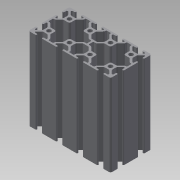
# Autodesk Inventor part: 25-5010
Saved by Autodesk Inventor 2013 (Build 170138000, 138)
## iProperties
Created: 2014-04-23
Part Number: 25-5010
Material: Generic
Document SubType Name: Modeling
Designer: Ross Bowman
Density: 1 g/cm^3
Engineer: Ross Bowman
Catalog Web Link: 8020.net
Vendor: 80/20 Inc.
Company: 80/20 Inc.
Author: Ross Bowman
Keywords: 80/20 , 8020 , T-Slot , Extrusion
Material: 6105-T5 Aluminum
Autodesk Inventor part; units mm, degrees
ref_plane "YZ Plane" through (0, 0, 0) normal (1, 0, 0) x (0, 1, 0)
ref_plane "XZ Plane" through (0, 0, 0) normal (0, 1, 0) x (-1, 0, 0)
ref_plane "XY Plane" through (0, 0, 0) normal (0, 0, 1) x (1, 0, 0)
sketch "Sketch1" plane through (0, 0, 0) normal (0, 0, 1) x (1, 0, 0)
  circle A0 centre (12.5003, -12.5001) radius 2.5
  circle A1 centre (37.5003, -12.5001) radius 2.5
  circle A2 centre (12.5003, 12.4999) radius 2.5
  circle A3 centre (37.5003, 12.4999) radius 2.5
  arc A4 (27.9491, 21.8456) -> (28.8746, 19.6112) centre (31.1091, 21.8456) ccw
  line L0 (32.3392, 16.1466) -> (28.8746, 19.6112)
  arc A5 (32.9878, 14.5807) -> (32.3392, 16.1466) centre (30.7732, 14.5807) ccw
  line L1 (32.9878, 10.1953) -> (32.9878, 14.5807)
  arc A6 (32.9878, 10.1953) -> (35.2024, 7.9807) centre (35.2024, 10.1953) ccw
  line L2 (39.5877, 7.9807) -> (35.2024, 7.9807)
  arc A7 (41.1537, 7.3321) -> (39.5877, 7.9807) centre (39.5877, 5.7661) ccw
  line L3 (44.6183, 3.8675) -> (41.1537, 7.3321)
  arc A8 (44.6183, 3.8675) -> (46.8527, 2.942) centre (46.8527, 6.102) ccw
  line L4 (47.1082, 2.942) -> (46.8527, 2.942)
  arc A9 (47.8588, 2.1914) -> (47.1082, 2.942) centre (47.1082, 2.1914) ccw
  line L5 (47.8588, -2.1939) -> (47.8588, 2.1914)
  arc A10 (47.1082, -2.9445) -> (47.8588, -2.1939) centre (47.1082, -2.1939) ccw
  line L6 (46.8527, -2.9445) -> (47.1082, -2.9445)
  arc A11 (46.8527, -2.9445) -> (44.6183, -3.8701) centre (46.8527, -6.1045) ccw
  line L7 (41.1537, -7.3346) -> (44.6183, -3.8701)
  arc A12 (39.5877, -7.9833) -> (41.1537, -7.3346) centre (39.5877, -5.7687) ccw
  line L8 (35.2024, -7.9833) -> (39.5877, -7.9833)
  arc A13 (35.2024, -7.9833) -> (32.9878, -10.1979) centre (35.2024, -10.1979) ccw
  line L9 (32.9878, -14.5832) -> (32.9878, -10.1979)
  arc A14 (32.3392, -16.1491) -> (32.9878, -14.5832) centre (30.7732, -14.5832) ccw
  line L10 (28.8746, -19.6137) -> (32.3392, -16.1491)
  arc A15 (28.8746, -19.6137) -> (27.9491, -21.8482) centre (31.1091, -21.8482) ccw
  line L11 (27.9491, -22.1036) -> (27.9491, -21.8482)
  arc A16 (27.1985, -22.8542) -> (27.9491, -22.1036) centre (27.1985, -22.1036) ccw
  line L12 (22.8132, -22.8542) -> (27.1985, -22.8542)
  arc A17 (22.0626, -22.1036) -> (22.8132, -22.8542) centre (22.8132, -22.1036) ccw
  line L13 (22.0626, -21.8482) -> (22.0626, -22.1036)
  arc A18 (22.0626, -21.8482) -> (21.137, -19.6137) centre (18.9026, -21.8482) ccw
  line L14 (17.6725, -16.1491) -> (21.137, -19.6137)
  arc A19 (17.0238, -14.5832) -> (17.6725, -16.1491) centre (19.2384, -14.5832) ccw
  line L15 (17.0238, -10.1979) -> (17.0238, -14.5832)
  arc A20 (17.0238, -10.1979) -> (14.8092, -7.9833) centre (14.8092, -10.1979) ccw
  line L16 (10.4239, -7.9833) -> (14.8092, -7.9833)
  arc A21 (8.8579, -7.3346) -> (10.4239, -7.9833) centre (10.4239, -5.7687) ccw
  line L17 (5.3934, -3.8701) -> (8.8579, -7.3346)
  arc A22 (5.3934, -3.8701) -> (3.1589, -2.9445) centre (3.1589, -6.1045) ccw
  line L18 (1.8176, -2.9445) -> (3.1589, -2.9445)
  arc A23 (1.067, -2.1939) -> (1.8176, -2.9445) centre (1.8176, -2.1939) ccw
  line L19 (1.067, 2.1914) -> (1.067, -2.1939)
  arc A24 (1.8176, 2.942) -> (1.067, 2.1914) centre (1.8176, 2.1914) ccw
  line L20 (3.1589, 2.942) -> (1.8176, 2.942)
  arc A25 (3.1589, 2.942) -> (5.3934, 3.8675) centre (3.1589, 6.102) ccw
  line L21 (8.8579, 7.3321) -> (5.3934, 3.8675)
  arc A26 (10.4239, 7.9807) -> (8.8579, 7.3321) centre (10.4239, 5.7661) ccw
  line L22 (14.8092, 7.9807) -> (10.4239, 7.9807)
  arc A27 (14.8092, 7.9807) -> (17.0238, 10.1953) centre (14.8092, 10.1953) ccw
  line L23 (17.0238, 14.5807) -> (17.0238, 10.1953)
  arc A28 (17.6725, 16.1466) -> (17.0238, 14.5807) centre (19.2384, 14.5807) ccw
  line L24 (21.137, 19.6112) -> (17.6725, 16.1466)
  arc A29 (21.137, 19.6112) -> (22.0626, 21.8456) centre (18.9026, 21.8456) ccw
  line L25 (22.0626, 22.1011) -> (22.0626, 21.8456)
  arc A30 (22.8132, 22.8517) -> (22.0626, 22.1011) centre (22.8132, 22.1011) ccw
  line L26 (27.1985, 22.8517) -> (22.8132, 22.8517)
  arc A31 (27.9491, 22.1011) -> (27.1985, 22.8517) centre (27.1985, 22.1011) ccw
  line L27 (27.9491, 21.8456) -> (27.9491, 22.1011)
  arc A32 (-2.9417, -21.8482) -> (-3.8673, -19.6137) centre (-6.1017, -21.8482) ccw
  line L28 (-7.0501, -16.4309) -> (-3.8673, -19.6137)
  arc A33 (-7.9756, -14.1965) -> (-7.0501, -16.4309) centre (-4.8156, -14.1965) ccw
  line L29 (-7.9756, -10.8104) -> (-7.9756, -14.1965)
  arc A34 (-7.0501, -8.5759) -> (-7.9756, -10.8104) centre (-4.8156, -10.8104) ccw
  line L30 (-3.8673, -5.3931) -> (-7.0501, -8.5759)
  arc A35 (-3.1559, -5.0984) -> (-3.8673, -5.3931) centre (-3.1559, -6.1045) ccw
  line L31 (3.1589, -5.0984) -> (-3.1559, -5.0984)
  arc A36 (3.8703, -5.3931) -> (3.1589, -5.0984) centre (3.1589, -6.1045) ccw
  line L32 (7.0531, -8.5759) -> (3.8703, -5.3931)
  arc A37 (7.9787, -10.8104) -> (7.0531, -8.5759) centre (4.8187, -10.8104) ccw
  line L33 (7.9787, -14.1965) -> (7.9787, -10.8104)
  arc A38 (7.0531, -16.4309) -> (7.9787, -14.1965) centre (4.8187, -14.1965) ccw
  line L34 (3.8703, -19.6137) -> (7.0531, -16.4309)
  arc A39 (3.8703, -19.6137) -> (2.9448, -21.8482) centre (6.1048, -21.8482) ccw
  line L35 (2.9448, -22.1036) -> (2.9448, -21.8482)
  arc A40 (2.1942, -22.8542) -> (2.9448, -22.1036) centre (2.1942, -22.1036) ccw
  line L36 (-2.1911, -22.8542) -> (2.1942, -22.8542)
  arc A41 (-2.9417, -22.1036) -> (-2.1911, -22.8542) centre (-2.1911, -22.1036) ccw
  line L37 (-2.9417, -21.8482) -> (-2.9417, -22.1036)
  circle A42 centre (-12.5003, -12.5001) radius 2.5
  circle A43 centre (-37.5003, -12.5001) radius 2.5
  arc A44 (-3.8673, 19.6112) -> (-2.9417, 21.8456) centre (-6.1017, 21.8456) ccw
  line L38 (-2.9417, 22.1011) -> (-2.9417, 21.8456)
  arc A45 (-2.1911, 22.8517) -> (-2.9417, 22.1011) centre (-2.1911, 22.1011) ccw
  line L39 (2.1942, 22.8517) -> (-2.1911, 22.8517)
  arc A46 (2.9448, 22.1011) -> (2.1942, 22.8517) centre (2.1942, 22.1011) ccw
  line L40 (2.9448, 21.8456) -> (2.9448, 22.1011)
  arc A47 (2.9448, 21.8456) -> (3.8703, 19.6112) centre (6.1048, 21.8456) ccw
  line L41 (7.0531, 16.4284) -> (3.8703, 19.6112)
  arc A48 (7.9787, 14.1939) -> (7.0531, 16.4284) centre (4.8187, 14.1939) ccw
  line L42 (7.9787, 10.8078) -> (7.9787, 14.1939)
  arc A49 (7.0531, 8.5734) -> (7.9787, 10.8078) centre (4.8187, 10.8078) ccw
  line L43 (3.8703, 5.3906) -> (7.0531, 8.5734)
  arc A50 (3.1589, 5.0959) -> (3.8703, 5.3906) centre (3.1589, 6.102) ccw
  line L44 (-3.1559, 5.0959) -> (3.1589, 5.0959)
  arc A51 (-3.8673, 5.3906) -> (-3.1559, 5.0959) centre (-3.1559, 6.102) ccw
  line L45 (-7.0501, 8.5734) -> (-3.8673, 5.3906)
  arc A52 (-7.9756, 10.8078) -> (-7.0501, 8.5734) centre (-4.8156, 10.8078) ccw
  line L46 (-7.9756, 14.1939) -> (-7.9756, 10.8078)
  arc A53 (-7.0501, 16.4284) -> (-7.9756, 14.1939) centre (-4.8156, 14.1939) ccw
  line L47 (-3.8673, 19.6112) -> (-7.0501, 16.4284)
  circle A54 centre (-12.5003, 12.4999) radius 2.5
  circle A55 centre (-37.5003, 12.4999) radius 2.5
  arc A56 (-28.8716, 19.6112) -> (-27.946, 21.8456) centre (-31.106, 21.8456) ccw
  line L48 (-27.946, 22.1011) -> (-27.946, 21.8456)
  arc A57 (-27.1954, 22.8517) -> (-27.946, 22.1011) centre (-27.1954, 22.1011) ccw
  line L49 (-22.8101, 22.8517) -> (-27.1954, 22.8517)
  arc A58 (-22.0595, 22.1011) -> (-22.8101, 22.8517) centre (-22.8101, 22.1011) ccw
  line L50 (-22.0595, 21.8456) -> (-22.0595, 22.1011)
  arc A59 (-22.0595, 21.8456) -> (-21.134, 19.6112) centre (-18.8995, 21.8456) ccw
  line L51 (-17.6694, 16.1466) -> (-21.134, 19.6112)
  arc A60 (-17.0208, 14.5807) -> (-17.6694, 16.1466) centre (-19.2354, 14.5807) ccw
  line L52 (-17.0208, 10.1953) -> (-17.0208, 14.5807)
  arc A61 (-17.0208, 10.1953) -> (-14.8062, 7.9807) centre (-14.8062, 10.1953) ccw
  line L53 (-10.4208, 7.9807) -> (-14.8062, 7.9807)
  arc A62 (-8.8549, 7.3321) -> (-10.4208, 7.9807) centre (-10.4208, 5.7661) ccw
  line L54 (-5.3903, 3.8675) -> (-8.8549, 7.3321)
  arc A63 (-5.3903, 3.8675) -> (-3.1559, 2.942) centre (-3.1559, 6.102) ccw
  line L55 (-1.8146, 2.942) -> (-3.1559, 2.942)
  arc A64 (-1.064, 2.1914) -> (-1.8146, 2.942) centre (-1.8146, 2.1914) ccw
  line L56 (-1.064, -2.1939) -> (-1.064, 2.1914)
  arc A65 (-1.8146, -2.9445) -> (-1.064, -2.1939) centre (-1.8146, -2.1939) ccw
  line L57 (-3.1559, -2.9445) -> (-1.8146, -2.9445)
  arc A66 (-3.1559, -2.9445) -> (-5.3903, -3.8701) centre (-3.1559, -6.1045) ccw
  line L58 (-8.8549, -7.3346) -> (-5.3903, -3.8701)
  arc A67 (-10.4208, -7.9833) -> (-8.8549, -7.3346) centre (-10.4208, -5.7687) ccw
  line L59 (-14.8062, -7.9833) -> (-10.4208, -7.9833)
  arc A68 (-14.8062, -7.9833) -> (-17.0208, -10.1979) centre (-14.8062, -10.1979) ccw
  line L60 (-17.0208, -14.5832) -> (-17.0208, -10.1979)
  arc A69 (-17.6694, -16.1491) -> (-17.0208, -14.5832) centre (-19.2354, -14.5832) ccw
  line L61 (-21.134, -19.6137) -> (-17.6694, -16.1491)
  arc A70 (-21.134, -19.6137) -> (-22.0595, -21.8482) centre (-18.8995, -21.8482) ccw
  line L62 (-22.0595, -22.1036) -> (-22.0595, -21.8482)
  arc A71 (-22.8101, -22.8542) -> (-22.0595, -22.1036) centre (-22.8101, -22.1036) ccw
  line L63 (-27.1954, -22.8542) -> (-22.8101, -22.8542)
  arc A72 (-27.946, -22.1036) -> (-27.1954, -22.8542) centre (-27.1954, -22.1036) ccw
  line L64 (-27.946, -21.8482) -> (-27.946, -22.1036)
  arc A73 (-27.946, -21.8482) -> (-28.8716, -19.6137) centre (-31.106, -21.8482) ccw
  line L65 (-32.3361, -16.1491) -> (-28.8716, -19.6137)
  arc A74 (-32.9848, -14.5832) -> (-32.3361, -16.1491) centre (-30.7702, -14.5832) ccw
  line L66 (-32.9848, -10.1979) -> (-32.9848, -14.5832)
  arc A75 (-32.9848, -10.1979) -> (-35.1994, -7.9833) centre (-35.1994, -10.1979) ccw
  line L67 (-39.5847, -7.9833) -> (-35.1994, -7.9833)
  arc A76 (-41.1506, -7.3346) -> (-39.5847, -7.9833) centre (-39.5847, -5.7687) ccw
  line L68 (-44.6152, -3.8701) -> (-41.1506, -7.3346)
  arc A77 (-44.6152, -3.8701) -> (-46.8497, -2.9445) centre (-46.8497, -6.1045) ccw
  line L69 (-47.1051, -2.9445) -> (-46.8497, -2.9445)
  arc A78 (-47.8557, -2.1939) -> (-47.1051, -2.9445) centre (-47.1051, -2.1939) ccw
  line L70 (-47.8557, 2.1914) -> (-47.8557, -2.1939)
  arc A79 (-47.1051, 2.942) -> (-47.8557, 2.1914) centre (-47.1051, 2.1914) ccw
  line L71 (-46.8497, 2.942) -> (-47.1051, 2.942)
  arc A80 (-46.8497, 2.942) -> (-44.6152, 3.8675) centre (-46.8497, 6.102) ccw
  line L72 (-41.1506, 7.3321) -> (-44.6152, 3.8675)
  arc A81 (-39.5847, 7.9807) -> (-41.1506, 7.3321) centre (-39.5847, 5.7661) ccw
  line L73 (-35.1994, 7.9807) -> (-39.5847, 7.9807)
  arc A82 (-35.1994, 7.9807) -> (-32.9848, 10.1953) centre (-35.1994, 10.1953) ccw
  line L74 (-32.9848, 14.5807) -> (-32.9848, 10.1953)
  arc A83 (-32.3361, 16.1466) -> (-32.9848, 14.5807) centre (-30.7702, 14.5807) ccw
  line L75 (-28.8716, 19.6112) -> (-32.3361, 16.1466)
  arc A84 (-30.3946, 21.1342) -> (-31.106, 22.8517) centre (-31.106, 21.8456) ccw
  line L76 (-30.3946, 21.1342) -> (-33.5774, 17.9514)
  arc A85 (-35.8119, 17.0259) -> (-33.5774, 17.9514) centre (-35.8119, 20.1859) ccw
  line L77 (-35.8119, 17.0259) -> (-39.198, 17.0259)
  arc A86 (-41.4324, 17.9514) -> (-39.198, 17.0259) centre (-39.198, 20.1859) ccw
  line L78 (-41.4324, 17.9514) -> (-44.6152, 21.1342)
  arc A87 (-43.9038, 22.8517) -> (-44.6152, 21.1342) centre (-43.9038, 21.8456) ccw
  line L79 (-43.9038, 22.8517) -> (-41.8233, 22.8517)
  arc A88 (-41.8233, 22.8517) -> (-41.8233, 24.9993) centre (-41.8233, 23.9255) ccw
  line L80 (-41.8233, 24.9993) -> (-48.003, 24.9993)
  arc A89 (-48.003, 24.9993) -> (-50.0034, 22.999) centre (-48.003, 22.999) ccw
  line L81 (-50.0034, 22.999) -> (-50.0034, 16.8193)
  arc A90 (-50.0034, 16.8193) -> (-47.8557, 16.8193) centre (-48.9296, 16.8193) ccw
  line L82 (-47.8557, 16.8193) -> (-47.8557, 18.8998)
  arc A91 (-46.1383, 19.6112) -> (-47.8557, 18.8998) centre (-46.8497, 18.8998) ccw
  line L83 (-46.1383, 19.6112) -> (-42.9555, 16.4284)
  arc A92 (-42.0299, 14.1939) -> (-42.9555, 16.4284) centre (-45.1899, 14.1939) ccw
  line L84 (-42.0299, 14.1939) -> (-42.0299, 10.8078)
  arc A93 (-42.9555, 8.5734) -> (-42.0299, 10.8078) centre (-45.1899, 10.8078) ccw
  line L85 (-42.9555, 8.5734) -> (-46.1383, 5.3906)
  arc A94 (-47.8557, 6.102) -> (-46.1383, 5.3906) centre (-46.8497, 6.102) ccw
  line L86 (-47.8557, 6.102) -> (-47.8557, 8.1825)
  arc A95 (-47.8557, 8.1825) -> (-50.0034, 8.1825) centre (-48.9296, 8.1825) ccw
  line L87 (-50.0034, 8.1825) -> (-50.0034, -8.185)
  arc A96 (-50.0034, -8.185) -> (-47.8557, -8.185) centre (-48.9296, -8.185) ccw
  line L88 (-47.8557, -8.185) -> (-47.8557, -6.1045)
  arc A97 (-46.1383, -5.3931) -> (-47.8557, -6.1045) centre (-46.8497, -6.1045) ccw
  line L89 (-46.1383, -5.3931) -> (-42.9555, -8.5759)
  arc A98 (-42.0299, -10.8104) -> (-42.9555, -8.5759) centre (-45.1899, -10.8104) ccw
  line L90 (-42.0299, -10.8104) -> (-42.0299, -14.1965)
  arc A99 (-42.9555, -16.4309) -> (-42.0299, -14.1965) centre (-45.1899, -14.1965) ccw
  line L91 (-42.9555, -16.4309) -> (-46.1383, -19.6137)
  arc A100 (-47.8557, -18.9023) -> (-46.1383, -19.6137) centre (-46.8497, -18.9023) ccw
  line L92 (-47.8557, -18.9023) -> (-47.8557, -16.8218)
  arc A101 (-47.8557, -16.8218) -> (-50.0034, -16.8218) centre (-48.9296, -16.8218) ccw
  line L93 (-50.0034, -16.8218) -> (-50.0034, -23.0015)
  arc A102 (-50.0034, -23.0015) -> (-48.003, -25.0019) centre (-48.003, -23.0015) ccw
  line L94 (-48.003, -25.0019) -> (-41.8233, -25.0019)
  arc A103 (-41.8233, -25.0019) -> (-41.8233, -22.8542) centre (-41.8233, -23.9281) ccw
  line L95 (-41.8233, -22.8542) -> (-43.9038, -22.8542)
  arc A104 (-44.6152, -21.1368) -> (-43.9038, -22.8542) centre (-43.9038, -21.8482) ccw
  line L96 (-44.6152, -21.1368) -> (-41.4324, -17.954)
  arc A105 (-39.198, -17.0284) -> (-41.4324, -17.954) centre (-39.198, -20.1884) ccw
  line L97 (-39.198, -17.0284) -> (-35.8119, -17.0284)
  arc A106 (-33.5774, -17.954) -> (-35.8119, -17.0284) centre (-35.8119, -20.1884) ccw
  line L98 (-33.5774, -17.954) -> (-30.3946, -21.1368)
  arc A107 (-31.106, -22.8542) -> (-30.3946, -21.1368) centre (-31.106, -21.8482) ccw
  line L99 (-31.106, -22.8542) -> (-33.1865, -22.8542)
  arc A108 (-33.1865, -22.8542) -> (-33.1865, -25.0019) centre (-33.1865, -23.9281) ccw
  line L100 (-33.1865, -25.0019) -> (-16.819, -25.0019)
  arc A109 (-16.819, -25.0019) -> (-16.819, -22.8542) centre (-16.819, -23.9281) ccw
  line L101 (-16.819, -22.8542) -> (-18.8995, -22.8542)
  arc A110 (-19.6109, -21.1368) -> (-18.8995, -22.8542) centre (-18.8995, -21.8482) ccw
  line L102 (-19.6109, -21.1368) -> (-16.4281, -17.954)
  arc A111 (-14.1937, -17.0284) -> (-16.4281, -17.954) centre (-14.1937, -20.1884) ccw
  line L103 (-14.1937, -17.0284) -> (-10.8076, -17.0284)
  arc A112 (-8.5731, -17.954) -> (-10.8076, -17.0284) centre (-10.8076, -20.1884) ccw
  line L104 (-8.5731, -17.954) -> (-5.3903, -21.1368)
  arc A113 (-6.1017, -22.8542) -> (-5.3903, -21.1368) centre (-6.1017, -21.8482) ccw
  line L105 (-6.1017, -22.8542) -> (-8.1822, -22.8542)
  arc A114 (-8.1822, -22.8542) -> (-8.1822, -25.0019) centre (-8.1822, -23.9281) ccw
  line L106 (-8.1822, -25.0019) -> (8.1853, -25.0019)
  arc A115 (8.1853, -25.0019) -> (8.1853, -22.8542) centre (8.1853, -23.9281) ccw
  line L107 (8.1853, -22.8542) -> (6.1048, -22.8542)
  arc A116 (5.3934, -21.1368) -> (6.1048, -22.8542) centre (6.1048, -21.8482) ccw
  line L108 (5.3934, -21.1368) -> (8.5762, -17.954)
  arc A117 (10.8106, -17.0284) -> (8.5762, -17.954) centre (10.8106, -20.1884) ccw
  line L109 (10.8106, -17.0284) -> (14.1967, -17.0284)
  arc A118 (16.4312, -17.954) -> (14.1967, -17.0284) centre (14.1967, -20.1884) ccw
  line L110 (16.4312, -17.954) -> (19.614, -21.1368)
  arc A119 (18.9026, -22.8542) -> (19.614, -21.1368) centre (18.9026, -21.8482) ccw
  line L111 (18.9026, -22.8542) -> (16.8221, -22.8542)
  arc A120 (16.8221, -22.8542) -> (16.8221, -25.0019) centre (16.8221, -23.9281) ccw
  line L112 (16.8221, -25.0019) -> (33.1896, -25.0019)
  arc A121 (33.1896, -25.0019) -> (33.1896, -22.8542) centre (33.1896, -23.9281) ccw
  line L113 (33.1896, -22.8542) -> (31.1091, -22.8542)
  arc A122 (30.3977, -21.1368) -> (31.1091, -22.8542) centre (31.1091, -21.8482) ccw
  line L114 (30.3977, -21.1368) -> (33.5804, -17.954)
  arc A123 (35.8149, -17.0284) -> (33.5804, -17.954) centre (35.8149, -20.1884) ccw
  line L115 (35.8149, -17.0284) -> (39.201, -17.0284)
  arc A124 (41.4355, -17.954) -> (39.201, -17.0284) centre (39.201, -20.1884) ccw
  line L116 (41.4355, -17.954) -> (44.6183, -21.1368)
  arc A125 (43.9068, -22.8542) -> (44.6183, -21.1368) centre (43.9068, -21.8482) ccw
  line L117 (43.9068, -22.8542) -> (41.8264, -22.8542)
  arc A126 (41.8264, -22.8542) -> (41.8264, -25.0019) centre (41.8264, -23.9281) ccw
  line L118 (41.8264, -25.0019) -> (48.0061, -25.0019)
  arc A127 (48.0061, -25.0019) -> (50.0064, -23.0015) centre (48.0061, -23.0015) ccw
  line L119 (50.0064, -23.0015) -> (50.0064, -16.8218)
  arc A128 (50.0064, -16.8218) -> (47.8588, -16.8218) centre (48.9326, -16.8218) ccw
  line L120 (47.8588, -16.8218) -> (47.8588, -18.9023)
  arc A129 (46.1413, -19.6137) -> (47.8588, -18.9023) centre (46.8527, -18.9023) ccw
  line L121 (46.1413, -19.6137) -> (42.9585, -16.4309)
  arc A130 (42.033, -14.1965) -> (42.9585, -16.4309) centre (45.193, -14.1965) ccw
  line L122 (42.033, -14.1965) -> (42.033, -10.8104)
  arc A131 (42.9585, -8.5759) -> (42.033, -10.8104) centre (45.193, -10.8104) ccw
  line L123 (42.9585, -8.5759) -> (46.1413, -5.3931)
  arc A132 (47.8588, -6.1045) -> (46.1413, -5.3931) centre (46.8527, -6.1045) ccw
  line L124 (47.8588, -6.1045) -> (47.8588, -8.185)
  arc A133 (47.8588, -8.185) -> (50.0064, -8.185) centre (48.9326, -8.185) ccw
  line L125 (50.0064, -8.185) -> (50.0064, 8.1825)
  arc A134 (50.0064, 8.1825) -> (47.8588, 8.1825) centre (48.9326, 8.1825) ccw
  line L126 (47.8588, 8.1825) -> (47.8588, 6.102)
  arc A135 (46.1413, 5.3906) -> (47.8588, 6.102) centre (46.8527, 6.102) ccw
  line L127 (46.1413, 5.3906) -> (42.9585, 8.5734)
  arc A136 (42.033, 10.8078) -> (42.9585, 8.5734) centre (45.193, 10.8078) ccw
  line L128 (42.033, 10.8078) -> (42.033, 14.1939)
  arc A137 (42.9585, 16.4284) -> (42.033, 14.1939) centre (45.193, 14.1939) ccw
  line L129 (42.9585, 16.4284) -> (46.1413, 19.6112)
  arc A138 (47.8588, 18.8998) -> (46.1413, 19.6112) centre (46.8527, 18.8998) ccw
  line L130 (47.8588, 18.8998) -> (47.8588, 16.8193)
  arc A139 (47.8588, 16.8193) -> (50.0064, 16.8193) centre (48.9326, 16.8193) ccw
  line L131 (50.0064, 16.8193) -> (50.0064, 22.999)
  arc A140 (50.0064, 22.999) -> (48.0061, 24.9993) centre (48.0061, 22.999) ccw
  line L132 (48.0061, 24.9993) -> (41.8264, 24.9993)
  arc A141 (41.8264, 24.9993) -> (41.8264, 22.8517) centre (41.8264, 23.9255) ccw
  line L133 (41.8264, 22.8517) -> (43.9068, 22.8517)
  arc A142 (44.6183, 21.1342) -> (43.9068, 22.8517) centre (43.9068, 21.8456) ccw
  line L134 (44.6183, 21.1342) -> (41.4355, 17.9514)
  arc A143 (39.201, 17.0259) -> (41.4355, 17.9514) centre (39.201, 20.1859) ccw
  line L135 (39.201, 17.0259) -> (35.8149, 17.0259)
  arc A144 (33.5804, 17.9514) -> (35.8149, 17.0259) centre (35.8149, 20.1859) ccw
  line L136 (33.5804, 17.9514) -> (30.3977, 21.1342)
  arc A145 (31.1091, 22.8517) -> (30.3977, 21.1342) centre (31.1091, 21.8456) ccw
  line L137 (31.1091, 22.8517) -> (33.1896, 22.8517)
  arc A146 (33.1896, 22.8517) -> (33.1896, 24.9993) centre (33.1896, 23.9255) ccw
  line L138 (33.1896, 24.9993) -> (16.8221, 24.9993)
  arc A147 (16.8221, 24.9993) -> (16.8221, 22.8517) centre (16.8221, 23.9255) ccw
  line L139 (16.8221, 22.8517) -> (18.9026, 22.8517)
  arc A148 (19.614, 21.1342) -> (18.9026, 22.8517) centre (18.9026, 21.8456) ccw
  line L140 (19.614, 21.1342) -> (16.4312, 17.9514)
  arc A149 (14.1967, 17.0259) -> (16.4312, 17.9514) centre (14.1967, 20.1859) ccw
  line L141 (14.1967, 17.0259) -> (10.8106, 17.0259)
  arc A150 (8.5762, 17.9514) -> (10.8106, 17.0259) centre (10.8106, 20.1859) ccw
  line L142 (8.5762, 17.9514) -> (5.3934, 21.1342)
  arc A151 (6.1048, 22.8517) -> (5.3934, 21.1342) centre (6.1048, 21.8456) ccw
  line L143 (6.1048, 22.8517) -> (8.1853, 22.8517)
  arc A152 (8.1853, 22.8517) -> (8.1853, 24.9993) centre (8.1853, 23.9255) ccw
  line L144 (8.1853, 24.9993) -> (-8.1822, 24.9993)
  arc A153 (-8.1822, 24.9993) -> (-8.1822, 22.8517) centre (-8.1822, 23.9255) ccw
  line L145 (-8.1822, 22.8517) -> (-6.1017, 22.8517)
  arc A154 (-5.3903, 21.1342) -> (-6.1017, 22.8517) centre (-6.1017, 21.8456) ccw
  line L146 (-5.3903, 21.1342) -> (-8.5731, 17.9514)
  arc A155 (-10.8076, 17.0259) -> (-8.5731, 17.9514) centre (-10.8076, 20.1859) ccw
  line L147 (-10.8076, 17.0259) -> (-14.1937, 17.0259)
  arc A156 (-16.4281, 17.9514) -> (-14.1937, 17.0259) centre (-14.1937, 20.1859) ccw
  line L148 (-16.4281, 17.9514) -> (-19.6109, 21.1342)
  arc A157 (-18.8995, 22.8517) -> (-19.6109, 21.1342) centre (-18.8995, 21.8456) ccw
  line L149 (-18.8995, 22.8517) -> (-16.819, 22.8517)
  arc A158 (-16.819, 22.8517) -> (-16.819, 24.9993) centre (-16.819, 23.9255) ccw
  line L150 (-16.819, 24.9993) -> (-33.1865, 24.9993)
  arc A159 (-33.1865, 24.9993) -> (-33.1865, 22.8517) centre (-33.1865, 23.9255) ccw
  line L151 (-33.1865, 22.8517) -> (-31.106, 22.8517)
  point P0 (0, 0)
  constraints: 304 end point, 304 point on circle, 160 centre point
extrude "Extrusion1" add sketch "Sketch1" against normal blind 100
body "Solid1"
